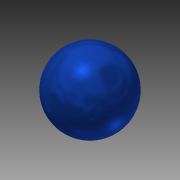
# Autodesk Inventor part: Blue Ball
Saved by Autodesk Inventor 2014 SP1 (Build 180222100, 222)
## iProperties
Created: 2014-01-23
Part Number: Blue Ball
Material: Generic
Document SubType Name: Modeling
Designer: jheinz37
Density: 1 g/cm^3
Appearance: Default
Author: jheinz37
Autodesk Inventor part; units mm, degrees
ref_plane "YZ Plane" through (0, 0, 0) normal (1, 0, 0) x (0, 1, 0)
ref_plane "XZ Plane" through (0, 0, 0) normal (0, 1, 0) x (-1, 0, 0)
ref_plane "XY Plane" through (0, 0, 0) normal (0, 0, 1) x (1, 0, 0)
sketch "Sketch1" plane through (0, 0, 0) normal (0, 0, 1) x (1, 0, 0)
  circle A0 centre (0, 0) radius 304.8
  line L0 (0, 304.8) -> (0, -304.8)
  dimension "d0" = 609.6
  dimension "d1" = 609.6
  constraints: 2 end point, 2 point on circle, 1 centre point, 1 coincident, 1 vertical
  measures "d0" diameter of A0
  measures "d1" distance of L0.start L0.end
revolve "Revolution1" add sketch "Sketch1" angle 360 about axis through (0, 304.8, 0) along (0, -1, 0) picked at (46.1254, 90.5263) contours A0 L0
body "Solid1"
